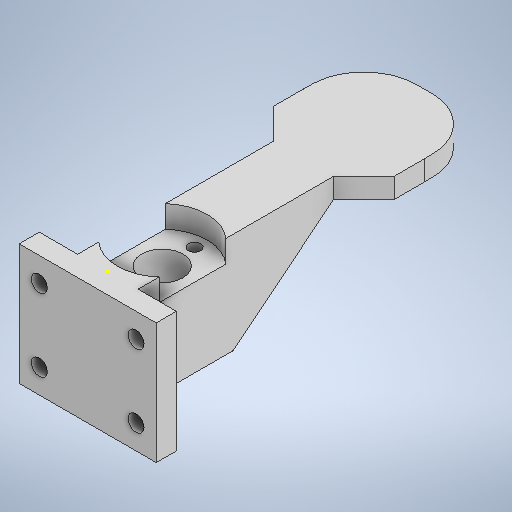
# Autodesk Inventor part: ActuatorV2
Saved by Autodesk Inventor 2025.1 (Build 291241000, 241)
## iProperties
Created: 2025-02-24
Part Number: ActuatorV2
Material: Generic
Document SubType Name: Modeling
Designer: 13156
Density: 1 g/cm^3
Appearance: Default
Author: 13156
Autodesk Inventor part; units mm, degrees
ref_plane "YZ Plane" through (0, 0, 0) normal (1, 0, 0) x (0, 1, 0)
ref_plane "XZ Plane" through (0, 0, 0) normal (0, 1, 0) x (-1, 0, 0)
ref_plane "XY Plane" through (0, 0, 0) normal (0, 0, 1) x (1, 0, 0)
sketch "Sketch1" plane through (0, 0, 0) normal (0, 0, 1) x (1, 0, 0)
  line L0 (-17, 15) -> (17, 15)
  line L1 (17, 15) -> (17, -15)
  line L2 (17, -15) -> (-17, -15)
  line L3 (-17, -15) -> (-17, 15)
  line L4 (0, 0) -> (0, 14.529) construction
  line L5 (0, 0) -> (24.325, 0) construction
  circle A0 centre (-12, 9) radius 2
  circle A1 centre (12, 9) radius 2
  circle A2 centre (12, -9) radius 2
  circle A3 centre (-12, -9) radius 2
  dimension "d0" = 30
  dimension "d1" = 34
  dimension "d2" = 4
  dimension "d3" = 24
  dimension "d4" = 24
  dimension "d5" = 18
  dimension "d6" = 18
  dimension "d7" = 5
  dimension "d8" = 6
  dimension "d9" = 5
  dimension "d10" = 5
  constraints: 12 end point, 4 centre point, 3 equal radius, 2 horizontal, 2 parallel, 1 perpendicular, 1 vertical, 2 other
  measures "d0" distance of L0.end L1.end
  measures "d1" distance of L0.start L0.end
  measures "d2" diameter of A0
  measures "d3" distance of A1.centre A0.centre
  measures "d4" distance of A2.centre A3.centre
  measures "d5" distance of A2.centre A1.centre
  measures "d6" distance of A3.centre A0.centre
  measures "d7" distance from line of L1 A2.centre
  measures "d8" distance from line of L2 A2.centre
  measures "d9" distance from line of L1 A1.centre
  measures "d10" distance from line of L3 A0.centre
extrude "Extrusion1" add sketch "Sketch1" along normal blind 5
sketch "Sketch2" plane through (-17, 15, 0) normal (0, 1, 0) x (1, 0, 0)
  line L0 (24.5, -5) -> (9.5, -5)
  line L1 (9.5, -5) -> (9.5, 48.5)
  line L2 (9.5, 48.5) -> (24.5, 48.5)
  line L3 (24.5, 48.5) -> (24.5, -5)
  circle A0 centre (17, 13.5) radius 5.125
  circle A1 centre (17, 21.5) radius 1.525
  circle A2 centre (17, 5.5) radius 1.525
  line L4 (17, -0.6376) -> (17, -5) construction
  line L5 (34, -5) -> (0, -5) projected
  circle A3 centre (17, 13.5) radius 11.15
  line L6 (34, 0) -> (0, 0) projected
  line L7 (17, 13.5) -> (17, 21.5) construction
  line L8 (17, 5.5) -> (17, 13.5) construction
  point P0 (17, 0)
  point P1 (17, 0)
  point P2 (17, 0)
  point P3 (9.5, 0)
  point P4 (24.5, 0)
  point P5 (17, 48.5)
  point P6 (17, 0)
  dimension "d13" = 10.25
  dimension "d14" = 3.05
  dimension "d15" = 3.05
  dimension "d16" = 8
  dimension "d17" = 8
  dimension "d18" = 22.3
  dimension "d19" = 18.5
  dimension "d24" = 15
  dimension "d25" = 7.5
  dimension "d48" = 48.5
  constraints: 14 end point, 5 midpoint, 4 centre point, 3 vertical, 2 parallel, 1 coincident, 1 collinear, 1 horizontal, 1 perpendicular, 1 other
  measures "d13" diameter of A0
  measures "d14" diameter of A2
  measures "d15" diameter of A1
  measures "d16" distance of L7.end A0.centre
  measures "d17" distance of A0.centre L8.start
  measures "d18" diameter of A3
  measures "d19" distance from line of A0.centre L5
  measures "d24" distance between parallel lines of L1 L3
  measures "d25" distance from line of L1 A0.centre
  measures "d48" distance from line of point (17, 0) L2
extrude "Extrusion2" add sketch "Sketch2" against normal blind 25 contours L0 L1 L6 L3 | L6 L1 A3 L3 | A3 L1 L3 | A3 L1 L2 L3
extrude "Extrusion3" cut sketch "Sketch2" against normal blind 5.5 contours A3 L1 L3 | L3 A3 | A3 L1
chamfer "Chamfer2" distance 3 angle 45 1 edges at (0, -10, 0)
sketch "Sketch3" plane through (-7.5, 15, -48.5) normal (0, 1, 0) x (1, 0, 0)
  point P0 (7.5, -48.5)
sketch "Sketch4" plane through (-7.5, 15, -48.5) normal (0, 1, 0) x (1, 0, 0)
  line L0 (22.5, 30) -> (-7.5, 30)
  line L1 (-7.5, 30) -> (-7.5, 0)
  line L2 (-7.5, 0) -> (22.5, 0)
  line L3 (22.5, 0) -> (22.5, 30)
  line L4 (15, 0) -> (0, 0) projected
  line L5 (7.5, 0) -> (7.5, 26.0274) construction
  point P0 (7.5, -48.5)
  dimension "d49" = 30
  dimension "d50" = 30
  constraints: 10 end point, 2 parallel, 1 collinear, 1 horizontal, 1 midpoint, 1 perpendicular, 1 vertical, 1 other
  measures "d49" distance of L2.end L0.start
  measures "d50" distance of L0.start L0.end
extrude "Extrusion4" add sketch "Sketch4" against normal blind 5
chamfer "Chamfer4" distance 25 distance2 20 1 edges at (0, -10, -48.5) measured on face at (0, -10, -48)
chamfer "Chamfer6" distance 7.5 angle 45 2 edges at (-15, 12.5, -48.5) (15, 12.5, -48.5)
fillet "Fillet7" radius 15 2 edges at (15, 12.5, -78.5) (-15, 12.5, -78.5) curvature continuous yes
equation "\"d4\" = d3"
equation "\"d6\" = d5"
equation "\"d9\" = d7"
equation "\"d10\" = d7"
equation "\"d15\" = d14"
equation "\"d17\" = d16"
equation "\"d25\" = 0.5 * d24"
body "Solid1"
